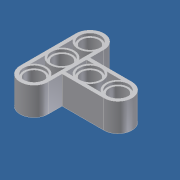
# Autodesk Inventor part: 5TM Beam
Saved by Autodesk Inventor 2016 (Build 200138000, 138)
## iProperties
Created: 2014-02-14
Part Number: 5TM Beam
Document SubType Name: Modeling
Designer: Jacob
Density: 1 g/cm^3
Material: Generic
Appearance: Default
Author: Jacob
Autodesk Inventor part; units mm, degrees
ref_plane "YZ Plane" through (0, 0, 0) normal (1, 0, 0) x (0, 1, 0)
ref_plane "XZ Plane" through (0, 0, 0) normal (0, 1, 0) x (-1, 0, 0)
ref_plane "XY Plane" through (0, 0, 0) normal (0, 0, 1) x (1, 0, 0)
sketch "Sketch1" plane through (0, 0, 0) normal (0, 0, 1) x (1, 0, 0)
  arc A0 (0, -4) -> (0, 4) centre (0, 0) ccw
  arc A1 (-12, 8) -> (-20, 8) centre (-16, 8) ccw
  arc A2 (-20, -8) -> (-12, -8) centre (-16, -8) ccw
  line L0 (-20, -8) -> (-20, 8)
  line L1 (0, 4) -> (-12, 4)
  line L2 (0, -4) -> (-12, -4)
  line L3 (-12, 8) -> (-12, 4)
  line L4 (-12, -4) -> (-12, -8)
  line L5 (-24.8, 0) -> (8.8, 0) projected
  line L6 (0, -16.8) -> (0, 16.8) projected
  dimension "d3" = 4
  dimension "d4" = 4
  dimension "d5" = 4
  dimension "d6" = 16
  dimension "d8" = 8
  dimension "d10" = 16
  dimension "d11" = 0
  dimension "d12" = 0
  dimension "d13" = 4
  constraints: 10 end point, 6 point on circle, 5 tangent, 3 centre point, 3 perpendicular, 2 parallel, 1 vertical
  measures "d3" radius of A0
  measures "d4" radius of A1
  measures "d5" radius of A2
  measures "d6" horizontal distance of A0.centre A1.centre
  measures "d8" vertical distance of A0.centre A1.centre
  measures "d10" distance of L0.start L0.end
  measures "d11" distance from line of A0.centre L5
  measures "d12" distance from line of A0.centre L6
  measures "d13" distance from line of L4 A2.centre
extrude "Extrusion1" add sketch "Sketch1" along normal blind 8
sketch "Sketch3" plane through (0, 0, 8) normal (0, 0, 1) x (1, 0, 0)
  arc A0 (0, -4) -> (0, 4) centre (0, 0) ccw projected
  circle A1 centre (0, 0) radius 2.5
  line L0 (-24.8, 0) -> (8.8, 0) projected
  circle A2 centre (-8, 0) radius 2.5
  dimension "d24" = 5
  dimension "d30" = 8
  constraints: 2 centre point, 1 coincident, 1 horizontal, 2 other
  measures "d24" diameter of A1
  measures "d30" distance of A1.centre A2.centre
extrude "Extrusion2" cut sketch "Sketch3" against normal through all
sketch "Sketch4" plane through (0, 0, 8) normal (0, 0, 1) x (1, 0, 0)
  arc A0 (-20, -8) -> (-12, -8) centre (-16, -8) ccw projected
  circle A1 centre (-16, -8) radius 2.5
  line L0 (0, -16.8) -> (0, 16.8) projected
  circle A2 centre (-16, 0) radius 2.5
  circle A3 centre (-16, 8) radius 2.5
  dimension "d34" = 5
  dimension "d40" = 8
  constraints: 3 centre point, 1 coincident, 1 vertical, 4 other
  measures "d34" diameter of A1
  measures "d40" distance of A1.centre A2.centre
extrude "Extrusion3" cut sketch "Sketch4" against normal through all
sketch "Sketch5" plane through (0, 0, 8) normal (0, 0, 1) x (1, 0, 0)
  circle A0 centre (-16, 8) radius 2.5 projected
  circle A1 centre (-16, 0) radius 2.5 projected
  circle A2 centre (-16, -8) radius 2.5 projected
  circle A3 centre (-8, 0) radius 2.5 projected
  circle A4 centre (0, 0) radius 2.5 projected
  arc A5 (-20, -8) -> (-12, -8) centre (-16, -8) ccw projected
  arc A6 (0, -4) -> (0, 4) centre (0, 0) ccw projected
  arc A7 (-12, 8) -> (-20, 8) centre (-16, 8) ccw projected
  circle A8 centre (-16, -8) radius 3
  circle A9 centre (-16, 0) radius 3
  circle A10 centre (-16, 8) radius 3
  circle A11 centre (-8, 0) radius 3
  circle A12 centre (0, 0) radius 3
  dimension "d44" = 6
  dimension "d45" = 6
  dimension "d46" = 6
  dimension "d47" = 6
  dimension "d48" = 6
  constraints: 5 centre point, 5 coincident
  measures "d44" diameter of A12
  measures "d45" diameter of A10
  measures "d46" diameter of A11
  measures "d47" diameter of A9
  measures "d48" diameter of A8
extrude "Extrusion4" cut sketch "Sketch5" against normal blind 0.8
sketch "Sketch6" plane through (0, 0, 0) normal (0, 0, -1) x (-1, 0, 0)
  circle A0 centre (16, 8) radius 2.5 projected
  circle A1 centre (16, 0) radius 2.5 projected
  circle A2 centre (16, -8) radius 2.5 projected
  circle A3 centre (8, 0) radius 2.5 projected
  circle A4 centre (0, 0) radius 2.5 projected
  arc A5 (12, -8) -> (20, -8) centre (16, -8) ccw projected
  arc A6 (20, 8) -> (12, 8) centre (16, 8) ccw projected
  arc A7 (0, 4) -> (0, -4) centre (0, 0) ccw projected
  circle A8 centre (8, 0) radius 3
  circle A9 centre (16, 8) radius 3
  circle A10 centre (0, 0) radius 3
  circle A11 centre (16, 0) radius 3
  circle A12 centre (16, -8) radius 3
  dimension "d52" = 6
  dimension "d53" = 6
  dimension "d54" = 6
  dimension "d55" = 6
  dimension "d56" = 6
  constraints: 5 centre point, 5 coincident
  measures "d52" diameter of A8
  measures "d53" diameter of A12
  measures "d54" diameter of A11
  measures "d55" diameter of A9
  measures "d56" diameter of A10
extrude "Extrusion5" cut sketch "Sketch6" against normal blind 0.8
sketch "Sketch7" plane through (0, 0, 8) normal (0, 0, 1) x (1, 0, 0)
  circle A0 centre (-16, -8) radius 3 projected
  circle A1 centre (-16, 0) radius 3 projected
  arc A2 (-20, -8) -> (-12, -8) centre (-16, -8) ccw projected
  arc A3 (-13, -6.1972) -> (-19, -6.1972) centre (-16, -8) ccw
  line L0 (-19, -1.8028) -> (-19, -6.1972)
  line L1 (-13, -1.8028) -> (-13, -6.1972)
  arc A4 (-19, -1.8028) -> (-13, -1.8028) centre (-16, 0) ccw
  line L2 (0, -16.8) -> (0, 16.8) projected
  arc A5 (-13, 1.8028) -> (-19, 1.8028) centre (-16, 0) ccw
  line L3 (-19, 6.1972) -> (-19, 1.8028)
  line L4 (-13, 6.1972) -> (-13, 1.8028)
  arc A6 (-19, 6.1972) -> (-13, 6.1972) centre (-16, 8) ccw
  dimension "d59" = 3.5
  dimension "d60" = 3.5
  dimension "d66" = 8
  constraints: 8 end point, 8 point on circle, 4 centre point, 4 tangent, 2 coincident, 1 vertical, 10 other
  measures "d59" radius of A4
  measures "d60" radius of A3
  measures "d66" distance of A4.centre A6.centre
extrude "Extrusion6" cut sketch "Sketch7" against normal through all contours A3 L0 A4 L1 | A5 L3 A6 L4
sketch "Sketch8" plane through (0, 0, 8) normal (0, 0, 1) x (1, 0, 0)
  line L0 (-13, -1.8028) -> (-13, -6.1972) projected
  circle A0 centre (-16, 0) radius 3 projected
  circle A1 centre (-8, 0) radius 3 projected
  arc A2 (0, -4) -> (0, 4) centre (0, 0) ccw projected
  line L1 (-12, 4) -> (0, 4) projected
  line L2 (-12, 8) -> (-12, 4) projected
  arc A3 (-1.8028, 3) -> (-1.8028, -3) centre (0, 0) ccw
  line L3 (-12, 3) -> (-12, -3)
  line L4 (-6.1972, -3) -> (-1.8028, -3)
  line L5 (-6.1972, 3) -> (-1.8028, 3)
  arc A4 (-9.8028, 3) -> (-9.8028, -3) centre (-8, 0) ccw
  arc A5 (-6.1972, -3) -> (-6.1972, 3) centre (-8, 0) ccw
  line L6 (-9.8028, 3) -> (-12, 3)
  line L7 (-9.8028, -3) -> (-12, -3)
  dimension "d72" = 3.5
  dimension "d73" = 3.5
  dimension "d74" = 3.5
  dimension "d75" = 2.1972
  constraints: 10 end point, 6 point on circle, 5 tangent, 3 centre point, 2 coincident, 2 collinear, 1 parallel, 1 perpendicular
  measures "d72" radius of A3
  measures "d73" radius of A5
  measures "d74" radius of A4
  measures "d75" distance of L7.start L3.end
extrude "Extrusion7" cut sketch "Sketch8" against normal through all contours A3 L4 A5 L5 | L6 A4 L7 L3
body "Solid1"
